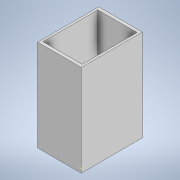
# Autodesk Inventor part: poerbankhållare
Saved by Autodesk Inventor 2022.1 (Build 261234020, 234B)
## iProperties
Created: 2021-11-06
Part Number: poerbankhållare
Material: Generic
Document SubType Name: Modeling
Designer: 46734
Density: 1 g/cm^3
Appearance: Default
Author: 46734
Autodesk Inventor part; units mm, degrees
ref_plane "YZ Plane" through (0, 0, 0) normal (1, 0, 0) x (0, 1, 0)
ref_plane "XZ Plane" through (0, 0, 0) normal (0, 1, 0) x (-1, 0, 0)
ref_plane "XY Plane" through (0, 0, 0) normal (0, 0, 1) x (1, 0, 0)
sketch "Sketch1" plane through (0, 0, 0) normal (0, 1, 0) x (-1, 0, 0)
  line L0 (0, 0) -> (50, 0)
  line L1 (50, 0) -> (50, -70)
  line L2 (50, -70) -> (0, -70)
  line L3 (0, -70) -> (0, 0)
  dimension "d0" = 50
  dimension "d1" = 70
  constraints: 8 end point, 2 parallel, 1 horizontal, 1 perpendicular
  measures "d0" distance of L1.end L2.end
  measures "d1" distance of L0.end L1.end
extrude "Extrusion1" add sketch "Sketch1" along normal blind 5
sketch "Sketch2" plane through (0, 5, 0) normal (0, 1, 0) x (1, 0, 0)
  line L0 (0, 0) -> (-50, 0)
  line L1 (-50, 70) -> (0, 70)
  line L2 (-2.5, 66.5) -> (-47.5, 66.5)
  line L3 (-47.5, 66.5) -> (-47.5, 3.5)
  line L4 (-47.5, 3.5) -> (-2.5, 3.5)
  line L5 (-2.5, 3.5) -> (-2.5, 66.5)
  line L6 (0, 0) -> (0, 70) projected
  line L7 (-50, 70) -> (-50, 0) projected
  line L8 (0, 70) -> (-50, 70) projected
  line L9 (-50, 0) -> (0, 0)
  line L10 (0, 0) -> (0, 70)
  line L11 (0, 70) -> (-50, 70)
  line L12 (-50, 70) -> (-50, 0)
  dimension "d22" = 63
  dimension "d24" = 45
  dimension "d25" = 2.5
  dimension "d27" = 3.5
  dimension "d28" = 50
  constraints: 20 end point, 3 horizontal, 3 parallel, 2 perpendicular, 1 vertical
  measures "d22" distance of L2.end L3.end
  measures "d24" distance of L3.end L4.end
  measures "d25" distance between parallel lines of L6 L5
  measures "d27" distance between parallel lines of L1 L2
  measures "d28" distance of L1.start L1.end
extrude "Extrusion2" add sketch "Sketch2" along normal blind 100
sketch "Sketch3" plane through (0, 5, 0) normal (0, 1, 0) x (1, 0, 0)
  point P0 (0, 0)
sketch "Sketch5" plane through (0, 5, 0) normal (0, 1, 0) x (1, 0, 0)
  line L0 (-47.5, 3.5) -> (-47.5, 66.5) projected
  line L1 (-2.5, 3.5) -> (-47.5, 3.5) projected
  line L2 (-2.5, 66.5) -> (-2.5, 3.5) projected
  line L3 (-47.5, 66.5) -> (-2.5, 66.5) projected
  point P0 (0, 0)
  point P1 (-44.5, 6.5)
  point P2 (-44.5, 63.5)
  point P3 (-5.5, 63.5)
  point P4 (-5.5, 6.5)
  dimension "d36" = 3
  dimension "d37" = 3
  dimension "d38" = 3
  dimension "d39" = 3
  dimension "d40" = 3
  dimension "d41" = 3
  dimension "d42" = 3
  dimension "d43" = 3
  measures "d36" distance from line of L0 point (-44.5, 6.5)
  measures "d37" distance from line of L1 point (-44.5, 6.5)
  measures "d38" distance from line of L2 point (-5.5, 6.5)
  measures "d39" distance from line of L1 point (-5.5, 6.5)
  measures "d40" distance from line of L2 point (-5.5, 63.5)
  measures "d41" distance from line of L3 point (-5.5, 63.5)
  measures "d42" distance from line of L3 point (-44.5, 63.5)
  measures "d43" distance from line of L0 point (-44.5, 63.5)
hole "Hole2" at (-44.5, 5, -6.5) at (-5.5, 5, -6.5) at (-5.5, 5, -63.5) at (-44.5, 5, -63.5) direction (0, -1, 0) diameter 3 end through all
body "Solid1"
